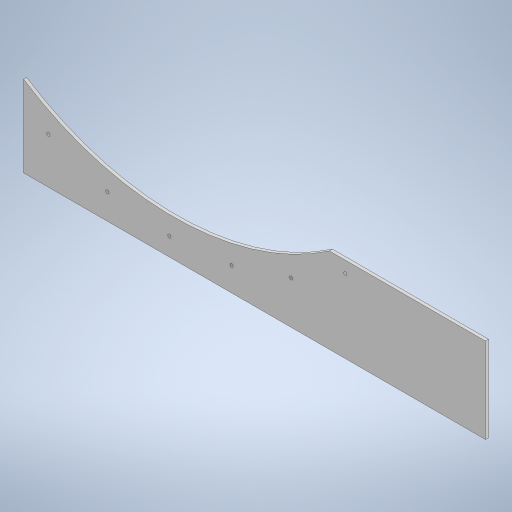
# Autodesk Inventor part: boundaryHalf2V1
Saved by Autodesk Inventor 2024.4 (Build 284460000, 460)
## iProperties
Created: 2025-11-05
Part Number: boundaryHalf2V1
Material: Generic
Document SubType Name: Modeling
Designer: jonas
Density: 1 g/cm^3
Appearance: Default
Author: jonas
Autodesk Inventor part; units mm, degrees
ref_plane "YZ Plane" through (0, 0, 0) normal (1, 0, 0) x (0, 1, 0)
ref_plane "XZ Plane" through (0, 0, 0) normal (0, 1, 0) x (-1, 0, 0)
ref_plane "XY Plane" through (0, 0, 0) normal (0, 0, 1) x (1, 0, 0)
sketch "Sketch2" plane through (0, 0, 0) normal (0, 1, 0) x (-1, 0, 0)
  line L0 (0, 329.241) -> (0, -329.241) construction
  line L1 (203.5937, 0) -> (-203.5937, 0) construction
  arc A0 (-250, -363.4133) -> (240, -370.0935) centre (0, 0) ccw
  line L2 (-500, -363.4133) -> (-500, -500)
  line L3 (-500, -500) -> (240, -500)
  line L4 (240, -500) -> (240, -370.0935)
  line L5 (-250, -363.4133) -> (-500, -363.4133)
  dimension "d0" = 500
  dimension "d2" = 500
  dimension "d3" = 441.1
  dimension "d5" = 363.4133
  dimension "d19" = 740
  constraints: 12 end point, 3 coincident, 3 perpendicular, 2 midpoint, 2 point on circle, 1 centre point, 1 horizontal, 1 vertical
  measures "d0" distance between parallel lines of L2 L0
  measures "d2" distance between parallel lines of L3 L1
  measures "d3" radius of A0
  measures "d5" distance between parallel lines of L1 L5
  measures "d19" distance between parallel lines of L4 L2
extrude "Extrusion1" add sketch "Sketch2" along normal blind 5
sketch "Sketch3" plane through (0, 0, 0) normal (0, -1, 0) x (1, 0, 0)
  line L0 (-200, -426.5386) -> (-105.4646, -459.1432) construction
  line L1 (-105.4646, -459.1432) -> (-6.1771, -471.0595) construction
  line L2 (-6.1771, -471.0595) -> (93.3887, -461.7508) construction
  line L3 (93.3887, -461.7508) -> (188.7465, -431.6364) construction
  line L4 (-200, -426.5386) -> (0, 0) construction
  line L5 (0, 0) -> (-105.4646, -459.1432) construction
  line L6 (0, 0) -> (-6.1771, -471.0595) construction
  line L7 (0, 0) -> (93.3887, -461.7508) construction
  line L8 (0, 0) -> (188.7465, -431.6364) construction
  line L9 (275.5998, -382.0732) -> (188.7465, -431.6364) construction
  line L10 (275.5998, -382.0732) -> (0, 0) construction
  line L11 (-240, -500) -> (-240, -370.0935) construction
  dimension "d8" = 471.1
  dimension "d9" = 100
  dimension "d10" = 40
  constraints: 22 end point, 9 equal length
  measures "d8" distance of L0.start L4.end
  measures "d9" distance of L0.start L0.end
  measures "d10" distance from line of L11 L0.start
hole "Hole1" at (-200, 0, -426.5386) at (-105.4646, 0, -459.1432) at (-6.1771, 0, -471.0595) at (93.3887, 0, -461.7508) at (188.7465, 0, -431.6364) at (275.5998, 0, -382.0732) direction (0, 1, 0) diameter 5 end through all
body "Solid1"
